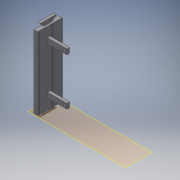
# Autodesk Inventor part: Bauteil3
Saved by Autodesk Inventor 2016 SP2 (Build 200236200, 236)
## iProperties
Created: 2018-06-21
Part Number: Bauteil3
Material: Generisch
Document SubType Name: Modeling
Designer: Nils
Density: 1 g/cm^3
Appearance: Vorgabe
Author: Nils
Autodesk Inventor part; units mm, degrees
ref_plane "YZ Plane" through (0, 0, 0) normal (1, 0, 0) x (0, 1, 0)
ref_plane "XZ Plane" through (0, 0, 0) normal (0, 1, 0) x (-1, 0, 0)
ref_plane "XY Plane" through (0, 0, 0) normal (0, 0, 1) x (1, 0, 0)
ref_plane "Arbeitsebene1" through (0, 0, 0) normal (0, 0, 1) x (1, 0, 0)
sketch "Skizze1" plane through (0, 0, 0) normal (0, 0, 1) x (1, 0, 0)
  line L0 (0, 1) -> (9, 1) projected
  line L1 (0, -14) -> (0, 1) projected
  line L2 (0, -45) -> (0, -30) projected
  line L3 (7.5, 0) -> (7.5, -17) projected
  line L4 (9, 0) -> (9, 1) projected
  line L5 (7.5, 0) -> (9, 0) projected
  line L6 (7.5, -17) -> (9, -17) projected
  line L7 (9, -17) -> (9, -17.5) projected
  line L8 (9, -17.5) -> (7.5, -19) projected
  line L9 (0, -14) -> (0, -30)
  line L10 (0, -45) -> (7.5, -45)
  line L11 (7.5, -45) -> (7.5, -19)
  point P0 (0, 0)
  constraints: 6 end point, 1 horizontal, 1 perpendicular, 1 vertical
extrude "Extrusion1" add sketch "Skizze1" along normal blind 138.8
sketch "Skizze2" plane through (0, -45, 0) normal (-1, 0, 0) x (0, 0, 1)
  line L0 (0, 46) -> (138.8, 46) construction
  line L1 (69.4, 46) -> (69.4, 0) construction
  line L2 (0, 0) -> (138.8, 0) construction
  line L3 (-8.0004, 39) -> (-0.0004, 31) projected
  line L4 (-8.0004, 7) -> (-8.0004, 39) projected
  line L5 (-0.0004, 15) -> (-8.0004, 7) projected
  circle A0 centre (-4.0004, 23) radius 1.75 projected
  line L6 (-0.0004, 31) -> (-0.0004, 15) projected
  line L7 (-8.0004, 39) -> (-0.0004, 31) projected
  line L8 (-8.0004, 7) -> (-8.0004, 39) projected
  line L9 (-0.0004, 15) -> (-8.0004, 7) projected
  line L10 (146.8002, 39.0002) -> (138.8002, 31.0002)
  line L11 (146.8, 7) -> (146.8, 39)
  line L12 (138.8002, 14.9998) -> (146.8002, 6.9998)
  circle A1 centre (142.8004, 23) radius 1.75
  line L13 (138.8, 31) -> (138.8, 15)
  line L14 (146.8002, 39.0002) -> (138.8002, 31.0002)
  line L15 (146.8, 7) -> (146.8, 39)
  line L16 (138.8002, 14.9998) -> (146.8002, 6.9998)
  line L17 (0, 0) -> (0, 46) construction
  line L18 (138.8, 46) -> (138.8, 0) construction
  point P0 (0, 45)
  point P1 (146.8004, 39)
  point P2 (138.8004, 31)
  point P3 (146.8004, 7)
  point P4 (138.8004, 15)
  constraints: 5 symmetric about line, 2 end point, 2 midpoint, 1 vertical, 2 other
extrude "Extrusion2" add sketch "Skizze2" against normal blind 4.4
sketch "Skizze3" plane through (0, -45, 0) normal (-1, 0, 0) x (0, 0, 1)
  circle A0 centre (-4, 23) radius 1.75 construction
  circle A1 centre (142.8, 23) radius 1.75 construction
  circle A2 centre (-4, 23) radius 3
  circle A3 centre (142.8, 23) radius 3
  point P0 (0, 45)
  dimension "d4" = 6
  dimension "d5" = 6
  constraints: 2 centre point, 2 coincident
  measures "d4" diameter of A2
  measures "d5" diameter of A3
extrude "Extrusion3" cut sketch "Skizze3" against normal blind 3.5
sketch "Skizze4" plane through (7.5, -45, 0) normal (1, 0, 0) x (0, 0, -1)
  line L0 (-138.8, 0) -> (-138.8, 26) projected
  line L1 (0, 26) -> (0, 0) projected
  line L2 (-138.8, 2) -> (0, 2)
  line L3 (0, 2) -> (0, 3)
  line L4 (0, 3) -> (-138.8, 3)
  line L5 (-138.8, 3) -> (-138.8, 2)
  line L6 (0, 0) -> (-138.8, 0) projected
  point P0 (0, 45)
  dimension "d8" = 1
  dimension "d9" = 2
  constraints: 8 end point, 2 parallel, 2 point on line, 1 horizontal, 1 perpendicular
  measures "d8" distance of L3.end L2.end
  measures "d9" distance between parallel lines of L6 L2
sketch "Skizze5" plane through (7.5, -45, 0) normal (1, 0, 0) x (0, 0, -1)
  line L0 (-138.8, 0) -> (-138.8, 26) construction
  line L1 (-138.8, 24) -> (0, 24) construction
  line L2 (0, 26) -> (0, 0) construction
  line L3 (-19.4, 24) -> (-29.4, 24)
  line L4 (-29.4, 24) -> (-29.4, 19)
  line L5 (-29.4, 19) -> (-19.4, 19)
  line L6 (-19.4, 19) -> (-19.4, 24)
  line L7 (-109.4, 24) -> (-119.4, 24)
  line L8 (-119.4, 24) -> (-119.4, 19)
  line L9 (-119.4, 19) -> (-109.4, 19)
  line L10 (-109.4, 19) -> (-109.4, 24)
  line L11 (-119.4, 19) -> (-138.8, 19) construction
  line L12 (-19.4, 19) -> (0, 19) construction
  line L13 (0, 26) -> (-138.8, 26) construction
  point P0 (0, 45)
  dimension "d10" = 10
  dimension "d11" = 5
  dimension "d12" = 5
  dimension "d13" = 10
  dimension "d14" = 80
  dimension "d15" = 2
  constraints: 22 end point, 7 point on line, 4 parallel, 3 horizontal, 3 perpendicular, 1 collinear
  measures "d10" distance of L4.end L5.end
  measures "d11" distance of L9.end L7.start
  measures "d12" distance of L5.end L3.start
  measures "d13" distance of L8.end L9.end
  measures "d14" distance between parallel lines of L10 L4
  measures "d15" distance between parallel lines of L13 L1
extrude "Extrusion4" add sketch "Skizze5" along normal blind 36.75
extrude "Extrusion5" add sketch "Skizze4" along normal blind 1 contours L0 L4 L1 L2
sketch "Skizze6" plane through (7.5, -26, 19.4) normal (0, -1, 0) x (1, 0, 0)
  circle A0 centre (31.75, 95) radius 1.75
  circle A1 centre (31.75, 5) radius 1.75
  line L0 (36.75, 100) -> (36.75, 90) projected
  line L1 (0, 90) -> (36.75, 90) projected
  line L2 (0, 10) -> (36.75, 10) projected
  line L3 (36.75, 10) -> (36.75, 0) projected
  point P0 (-7.5, -19.4)
  dimension "d20" = 3.5
  dimension "d21" = 3.5
  dimension "d22" = 5
  dimension "d23" = 5
  dimension "d24" = 5
  dimension "d25" = 5
  constraints: 2 centre point
  measures "d20" diameter of A0
  measures "d21" diameter of A1
  measures "d22" distance from line of L0 A0.centre
  measures "d23" distance from line of L1 A0.centre
  measures "d24" distance from line of L2 A1.centre
  measures "d25" distance from line of L3 A1.centre
extrude "Extrusion6" cut sketch "Skizze6" against normal blind 10
sketch "Skizze7" plane through (7.5, -21, 29.4) normal (0, 1, 0) x (1, 0, 0)
  circle A0 centre (31.75, 5) radius 1.75 construction
  circle A1 centre (31.75, -85) radius 1.75 construction
  circle A2 centre (31.75, 5) radius 1.75 projected
  line L0 (30.0757, 2.1) -> (28.4014, 5)
  line L1 (28.4014, 5) -> (30.0757, 7.9)
  line L2 (30.0757, 7.9) -> (33.4243, 7.9)
  line L3 (33.4243, 7.9) -> (35.0986, 5)
  line L4 (35.0986, 5) -> (33.4243, 2.1)
  line L5 (33.4243, 2.1) -> (30.0757, 2.1)
  circle A3 centre (31.75, -85) radius 1.75 projected
  line L6 (28.4014, -85) -> (30.0757, -82.1)
  line L7 (30.0757, -82.1) -> (33.4243, -82.1)
  line L8 (33.4243, -82.1) -> (35.0986, -85)
  line L9 (35.0986, -85) -> (33.4243, -87.9)
  line L10 (33.4243, -87.9) -> (30.0757, -87.9)
  line L11 (30.0757, -87.9) -> (28.4014, -85)
  point P0 (-7.5, 29.4)
  dimension "d28" = 5.8
  dimension "d29" = 5.8
  constraints: 24 end point, 2 coincident, 2 horizontal, 26 other
  measures "d28" distance between parallel lines of L0 L3
  measures "d29" distance between parallel lines of L10 L7
extrude "Extrusion7" cut sketch "Skizze7" against normal blind 2.5
equation "\"d12\" = d11"
equation "\"d13\" = d10"
equation "\"d21\" = d20"
equation "\"d23\" = d22"
equation "\"d24\" = d22"
equation "\"d25\" = d22"
equation "\"d29\" = d28"
